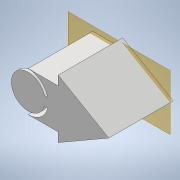
# Autodesk Inventor part: Wire_Clossing_3
Saved by Autodesk Inventor 2022.3 (Build 263350000, 350)
## iProperties
Created: 2023-05-23
Part Number: Wire_Clossing_3
Material: Generic
Document SubType Name: Modeling
Designer: Manuel Hueso Béjar
Density: 1 g/cm^3
Appearance: Default
Author: Manuel Hueso Béjar
Autodesk Inventor part; units mm, degrees
ref_plane "YZ Plane" through (0, 0, 0) normal (1, 0, 0) x (0, 1, 0)
ref_plane "XZ Plane" through (0, 0, 0) normal (0, 1, 0) x (-1, 0, 0)
ref_plane "XY Plane" through (0, 0, 0) normal (0, 0, 1) x (1, 0, 0)
sketch "Sketch1" plane through (0, 0, 0) normal (0, 0, 1) x (1, 0, 0)
  arc A0 (-20.1728, 11.5) -> (-26.235, 13) centre (-26.235, 0) ccw projected
  line L0 (-5.235, 11.5) -> (-20.1728, 11.5) projected
  line L1 (-5.235, 16.4372) -> (-5.235, 11.5) projected
  line L2 (23.235, 0) -> (-5.235, 16.4372) projected
  line L3 (-5.235, -16.4372) -> (23.235, 0) projected
  line L4 (-5.235, -11.5) -> (-5.235, -16.4372) projected
  line L5 (-20.1728, -11.5) -> (-5.235, -11.5) projected
  arc A1 (-26.235, -13) -> (-20.1728, -11.5) centre (-26.235, 0) ccw projected
  line L6 (-6.735, -13) -> (-26.235, -13) projected
  line L7 (-6.735, -19.0353) -> (-6.735, -13) projected
  line L8 (26.235, 0) -> (-6.735, -19.0353) projected
  line L9 (-6.735, 19.0353) -> (26.235, 0) projected
  line L10 (-6.735, 13) -> (-6.735, 19.0353) projected
  line L11 (-26.235, 13) -> (-6.735, 13) projected
  point P0 (0, 0)
extrude "Extrusion1" add sketch "Sketch1" along normal up to surface (42 mm away)
ref_plane "Work Plane1" through (-6.5, 0, 2) normal (0, 0, 1) x (1, 0, 0)
sketch "Sketch2" plane through (-26.235, -13, 42) normal (0, 0, 1) x (1, 0, 0)
  circle A0 centre (0, 13) radius 4.1 projected
  line L0 (6.0622, 1.5) -> (21, 1.5) projected
  line L1 (21, 1.5) -> (21, -3.4372) projected
  line L2 (21, -3.4372) -> (49.4701, 13) projected
  line L3 (49.4701, 13) -> (21, 29.4372) projected
  line L4 (21, 29.4372) -> (21, 24.5) projected
  line L5 (21, 24.5) -> (6.0622, 24.5) projected
  arc A1 (12, 18) -> (6.0622, 24.5) centre (0, 13) ccw projected
  line L6 (12, 18) -> (13.6491, 18) projected
  line L7 (13.6491, 18) -> (15.6491, 20) projected
  line L8 (15.6491, 20) -> (15.6491, 16) projected
  line L9 (15.6491, 16) -> (10.583, 16) projected
  arc A2 (10.583, 16) -> (10.583, 10) centre (0, 13) ccw projected
  line L10 (10.583, 10) -> (15.6491, 10) projected
  line L11 (15.6491, 10) -> (15.6491, 6) projected
  line L12 (15.6491, 6) -> (13.6491, 8) projected
  line L13 (13.6491, 8) -> (12, 8) projected
  arc A3 (6.0622, 1.5) -> (12, 8) centre (0, 13) ccw projected
  circle A4 centre (24.5, 13) radius 7 projected
  line L14 (15.8491, 5.5172) -> (15.8491, 10.2)
  line L15 (15.8491, 10.2) -> (10.4307, 10.2)
  arc A5 (10.4307, 15.8) -> (10.4307, 10.2) centre (0, 13) ccw
  line L16 (10.4307, 15.8) -> (15.8491, 15.8)
  line L17 (15.8491, 15.8) -> (15.8491, 20.4828)
  line L18 (15.8491, 20.4828) -> (13.5663, 18.2)
  line L19 (13.5663, 18.2) -> (12.1326, 18.2)
  arc A6 (12.1326, 18.2) -> (6.8228, 24.3) centre (0, 13) ccw
  line L20 (6.8228, 24.3) -> (21.2, 24.3)
  line L21 (21.2, 24.3) -> (21.2, 29.0908)
  line L22 (21.2, 29.0908) -> (49.0701, 13)
  line L23 (49.0701, 13) -> (21.2, -3.0908)
  line L24 (21.2, -3.0908) -> (21.2, 1.7)
  line L25 (21.2, 1.7) -> (6.8228, 1.7)
  arc A7 (6.8228, 1.7) -> (12.1326, 7.8) centre (0, 13) ccw
  line L26 (12.1326, 7.8) -> (13.5663, 7.8)
  line L27 (13.5663, 7.8) -> (15.8491, 5.5172)
  line L28 (16.8491, 11.2) -> (16.8491, 3.1029)
  line L29 (16.8491, 3.1029) -> (13.1521, 6.8)
  line L30 (13.1521, 6.8) -> (12.775, 6.8)
  arc A8 (9.775, 2.7) -> (12.775, 6.8) centre (0, 13) ccw
  line L31 (9.775, 2.7) -> (22.2, 2.7)
  line L32 (22.2, 2.7) -> (22.2, -1.3587)
  line L33 (22.2, -1.3587) -> (47.0701, 13)
  line L34 (47.0701, 13) -> (22.2, 27.3587)
  line L35 (22.2, 27.3587) -> (22.2, 23.3)
  line L36 (22.2, 23.3) -> (9.775, 23.3)
  arc A9 (12.775, 19.2) -> (9.775, 23.3) centre (0, 13) ccw
  line L37 (12.775, 19.2) -> (13.1521, 19.2)
  line L38 (13.1521, 19.2) -> (16.8491, 22.8971)
  line L39 (16.8491, 22.8971) -> (16.8491, 14.8)
  line L40 (16.8491, 14.8) -> (9.6333, 14.8)
  arc A10 (9.6333, 14.8) -> (9.6333, 11.2) centre (0, 13) ccw
  line L41 (9.6333, 11.2) -> (16.8491, 11.2)
  line L42 (15.6491, 10) -> (16.8491, 10)
  line L43 (16.8491, 10) -> (16.8491, 11.2)
  line L44 (16.8491, 11.2) -> (15.6491, 11.2)
  line L45 (15.6491, 11.2) -> (15.6491, 10)
  line L46 (15.6491, 16) -> (16.8491, 16)
  line L47 (16.8491, 16) -> (16.8491, 14.8)
  line L48 (16.8491, 14.8) -> (15.6491, 14.8)
  line L49 (15.6491, 14.8) -> (15.6491, 16)
  line L50 (6.8228, 1.7) -> (6.8228, 1.5)
  line L51 (21, 1.5) -> (6.0622, 1.5) projected
  line L52 (6.8228, 24.3) -> (6.8228, 24.5)
  line L53 (6.0622, 24.5) -> (21, 24.5) projected
  line L54 (16.8491, 3.1029) -> (16.8491, 1.5)
  line L55 (16.8491, 1.5) -> (6.8228, 1.5)
  line L56 (16.8491, 22.8971) -> (16.8491, 24.5)
  line L57 (16.8491, 24.5) -> (6.8228, 24.5)
  point P0 (26.235, 13)
  point P1 (6.8228, 24.5)
  point P2 (15.8491, 16)
  point P3 (15.8491, 10)
  point P4 (6.8228, 1.5)
  dimension "d2" = 0.2
  dimension "d3" = 1
  constraints: 84 end point, 12 point on circle, 8 point on line, 6 centre point, 4 parallel, 4 perpendicular, 2 horizontal, 1 collinear, 32 other
  measures "d2" distance between parallel lines of L11 L14
  measures "d3" distance between parallel lines of L14 L28
ref_plane "Work Plane2" through (-37.235, -16.4372, 2) normal (0, 0, 1) x (1, 0, 0)
extrude "Extrusion2" add sketch "Sketch2" against normal up to surface (40 mm away) contours L50 L25 L54 L0 | A7 L26 L27 L14 L42 L28 L29 L30 A8 L31 L54 L25 | L31 A8 L30 L29 L54 | L56 L20 L52 L5 | L17 L18 L19 A6 L20 L56 L36 A9 L37 L38 L39 L46 | L56 L38 L37 A9 L36
ref_plane "Work Plane3" through (-6.5, 0, 2) normal (0, 0, 1) x (1, 0, 0)
sketch "Sketch3" plane through (-26.235, -13, 42) normal (0, 0, 1) x (1, 0, 0)
  circle A0 centre (0, 13) radius 4.1 projected
  line L0 (6.0622, 1.5) -> (21, 1.5) projected
  line L1 (21, 1.5) -> (21, -3.4372) projected
  line L2 (21, -3.4372) -> (49.4701, 13) projected
  line L3 (49.4701, 13) -> (21, 29.4372) projected
  line L4 (21, 29.4372) -> (21, 24.5) projected
  line L5 (21, 24.5) -> (6.0622, 24.5) projected
  arc A1 (12, 18) -> (6.0622, 24.5) centre (0, 13) ccw projected
  line L6 (12, 18) -> (13.6491, 18) projected
  line L7 (13.6491, 18) -> (15.6491, 20) projected
  line L8 (15.6491, 20) -> (15.6491, 16) projected
  line L9 (15.6491, 16) -> (10.583, 16) projected
  arc A2 (10.583, 16) -> (10.583, 10) centre (0, 13) ccw projected
  line L10 (10.583, 10) -> (15.6491, 10) projected
  line L11 (15.6491, 10) -> (15.6491, 6) projected
  line L12 (15.6491, 6) -> (13.6491, 8) projected
  line L13 (13.6491, 8) -> (12, 8) projected
  arc A3 (6.0622, 1.5) -> (12, 8) centre (0, 13) ccw projected
  circle A4 centre (24.5, 13) radius 7 projected
  line L14 (16.8491, 1.5) -> (15.6491, 1.5)
  line L15 (15.6491, 1.5) -> (15.6491, 10)
  line L16 (15.6491, 10) -> (16.8491, 10)
  line L17 (16.8491, 10) -> (16.8491, 1.5)
  line L18 (16.8491, 24.5) -> (16.8491, 16) projected
  line L19 (15.6491, 16) -> (16.8491, 16)
  line L20 (16.8491, 16) -> (16.8491, 24.5)
  line L21 (16.8491, 24.5) -> (15.6491, 24.5)
  line L22 (15.6491, 24.5) -> (15.6491, 16)
  line L23 (12, 8) -> (15.6491, 8)
  line L24 (15.6491, 8) -> (15.6491, 10)
  line L25 (15.6491, 10) -> (12, 10)
  line L26 (12, 10) -> (12, 8)
  line L27 (12, 18) -> (15.6491, 18)
  line L28 (15.6491, 18) -> (15.6491, 16)
  line L29 (15.6491, 16) -> (12, 16)
  line L30 (12, 16) -> (12, 18)
  arc A5 (10.583, 16) -> (10.583, 10) centre (0, 13) ccw projected
  line L31 (10.583, 16) -> (12.6491, 16) projected
  arc A6 (12.6491, 16) -> (12.6491, 10) centre (0, 13) ccw projected
  line L32 (12.6491, 10) -> (10.583, 10) projected
  point P0 (26.235, 13)
  constraints: 32 end point, 8 parallel, 4 horizontal, 4 perpendicular
ref_plane "Work Plane4" through (-14.235, -7, 22) normal (0, 0, 1) x (1, 0, 0)
extrude "Extrusion3" add sketch "Sketch3" against normal up to surface (20 mm away) contours A3 L13 L12 L15 L0 | L15 L11 L16 L17 L0 | A6 L10 L11 L23 L13 | L5 L22 L7 L6 A1 | L12 L23 L11 | L5 L18 L19 L8 L22 | L6 L27 L8 L9 A6 | L8 L27 L7
ref_plane "Work Plane5" through (-6.5, 0, 2) normal (0, 0, 1) x (1, 0, 0)
sketch "Sketch4" plane through (-26.235, -13, 42) normal (0, 0, 1) x (1, 0, 0)
  circle A0 centre (0, 13) radius 4.1 projected
  line L0 (6.0622, 1.5) -> (21, 1.5) projected
  line L1 (21, 1.5) -> (21, -3.4372) projected
  line L2 (21, -3.4372) -> (49.4701, 13) projected
  line L3 (49.4701, 13) -> (21, 29.4372) projected
  line L4 (21, 29.4372) -> (21, 24.5) projected
  line L5 (21, 24.5) -> (6.0622, 24.5) projected
  arc A1 (12, 18) -> (6.0622, 24.5) centre (0, 13) ccw projected
  line L6 (12, 18) -> (13.6491, 18) projected
  line L7 (13.6491, 18) -> (15.6491, 20) projected
  line L8 (15.6491, 20) -> (15.6491, 16) projected
  line L9 (15.6491, 16) -> (10.583, 16) projected
  arc A2 (10.583, 16) -> (10.583, 10) centre (0, 13) ccw projected
  line L10 (10.583, 10) -> (15.6491, 10) projected
  line L11 (15.6491, 10) -> (15.6491, 6) projected
  line L12 (15.6491, 6) -> (13.6491, 8) projected
  line L13 (13.6491, 8) -> (12, 8) projected
  arc A3 (6.0622, 1.5) -> (12, 8) centre (0, 13) ccw projected
  circle A4 centre (24.5, 13) radius 7 projected
  point P0 (26.235, 13)
extrude "Extrusion4" add sketch "Sketch4" against normal blind 2 contours A0 | A3 L13 L12 L11 L10 A2 L9 L8 L7 L6 A1 L5 L4 L3 L2 L1 L0 | A4
body "Solid1"
